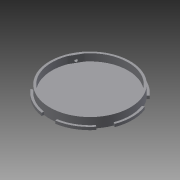
# Autodesk Inventor part: base
Saved by Autodesk Inventor 2015 (Build 190159000, 159)
## iProperties
Created: 2019-10-01
Part Number: base
Material: Generic
Document SubType Name: Modeling
Designer: gabri
Density: 1 g/cm^3
Appearance: Default
Author: gabri
Autodesk Inventor part; units mm, degrees
ref_plane "YZ Plane" through (0, 0, 0) normal (1, 0, 0) x (0, 1, 0)
sketch "Sketch1" plane through (0, 0, 0) normal (0, 0, 1) x (1, 0, 0)
  line L0 (-49.0069, -18.1093) -> (-50.1652, -19.0624) projected
  arc A0 (-50.1652, -19.0624) -> (-31.7077, -29.6283) centre (-27, 0) ccw projected
  line L1 (-31.7077, -29.6283) -> (-31.4723, -28.1469) projected
  arc A1 (-31.4723, -28.1469) -> (-22.3204, -28.1132) centre (-27, 0) ccw projected
  line L2 (-22.3204, -28.1132) -> (-22.0741, -29.5928) projected
  arc A2 (-22.0741, -29.5928) -> (-3.6949, -18.8911) centre (-27, 0) ccw projected
  line L3 (-3.6949, -18.8911) -> (-4.8602, -17.9466) projected
  arc A3 (-4.8602, -17.9466) -> (-0.3135, -10.0039) centre (-27, 0) ccw projected
  line L4 (-0.3135, -10.0039) -> (1.0911, -10.5304) projected
  arc A4 (1.0911, -10.5304) -> (1.0127, 10.7372) centre (-27, 0) ccw projected
  line L5 (1.0127, 10.7372) -> (-0.3879, 10.2004) projected
  arc A5 (-0.3879, 10.2004) -> (-4.9931, 18.1093) centre (-27, 0) ccw projected
  line L6 (-4.9931, 18.1093) -> (-3.8348, 19.0624) projected
  arc A6 (-3.8348, 19.0624) -> (-22.2923, 29.6283) centre (-27, 0) ccw projected
  line L7 (-22.2923, 29.6283) -> (-22.5277, 28.1469) projected
  arc A7 (-22.5277, 28.1469) -> (-31.6796, 28.1132) centre (-27, 0) ccw projected
  line L8 (-31.6796, 28.1132) -> (-31.9259, 29.5928) projected
  arc A8 (-31.9259, 29.5928) -> (-50.3051, 18.8911) centre (-27, 0) ccw projected
  line L9 (-50.3051, 18.8911) -> (-49.1398, 17.9466) projected
  arc A9 (-49.1398, 17.9466) -> (-53.6865, 10.0039) centre (-27, 0) ccw projected
  line L10 (-53.6865, 10.0039) -> (-55.0911, 10.5304) projected
  arc A10 (-55.0911, 10.5304) -> (-55.0127, -10.7372) centre (-27, 0) ccw projected
  line L11 (-55.0127, -10.7372) -> (-53.6121, -10.2004) projected
  arc A11 (-53.6121, -10.2004) -> (-49.0069, -18.1093) centre (-27, 0) ccw projected
  line L12 (-0.0417, 1.5) -> (1, 1.5) projected
  line L13 (1, 1.5) -> (1, -1.5) projected
  line L14 (1, -1.5) -> (-0.0417, -1.5) projected
  arc A12 (-53.9583, -1.5) -> (-0.0417, -1.5) centre (-27, 0) ccw projected
  line L15 (-53.9583, -1.5) -> (-55, -1.5) projected
  line L16 (-55, -1.5) -> (-55, 1.5) projected
  line L17 (-55, 1.5) -> (-53.9583, 1.5) projected
  arc A13 (-0.0417, 1.5) -> (-53.9583, 1.5) centre (-27, 0) ccw projected
  circle A14 centre (-27, 0) radius 30
  point P0 (0, 0)
  constraints: 1 centre point, 1 coincident, 1 concentric
extrude "Extrusion1" add sketch "Sketch1" along normal blind 2 contours A11 L11 A10 L10 A9 L9 A8 L8 A7 L7 A6 L6 A5 L5 A4 L4 A3 L3 A2 L2 A1 L1 A0 L0 | L12 L13 L14 A12 L15 L16 L17 A13
sketch "Sketch2" plane through (0, 0, 2) normal (0, 0, 1) x (1, 0, 0)
  arc A0 (-53.9583, -1.5) -> (-0.0417, -1.5) centre (-27, 0) ccw projected
  arc A1 (-0.0417, 1.5) -> (-53.9583, 1.5) centre (-27, 0) ccw projected
  circle A2 centre (-27, 0) radius 28.5 projected
  circle A3 centre (-27, 0) radius 27
  circle A4 centre (-27, 0) radius 28.5
  point P0 (0, 0)
  constraints: 2 centre point, 2 coincident, 2 concentric
ref_plane "Work Plane1" through (-31.9259, 28.1132, 7) normal (0, 0, 1) x (1, 0, 0)
extrude "Extrusion2" add sketch "Sketch2" along normal up to surface (5 mm away)
sketch "Sketch3" plane through (-27, 0, 2) normal (0, 0, 1) x (1, 0, 0)
  circle A0 centre (0, 0) radius 27 projected
  circle A1 centre (0, 0) radius 28.5 projected
  line L0 (-23.3051, 18.8911) -> (-28.0911, 10.5304) projected
  line L1 (-28.0911, 10.5304) -> (-26.6865, 10.0039) projected
  arc A2 (-22.1398, 17.9466) -> (-26.6865, 10.0039) centre (0, 0) ccw projected
  line L2 (-22.1398, 17.9466) -> (-23.3051, 18.8911) projected
  line L3 (-22.1398, 17.9466) -> (-20.9746, 17.002)
  line L4 (-26.6865, 10.0039) -> (-25.282, 9.4774)
  line L5 (-20.9746, 17.002) -> (-25.282, 9.4774)
  point P0 (27, 0)
  constraints: 6 end point, 2 collinear, 2 point on circle
ref_plane "Work Plane2" through (-55.0911, 10.0039, 7) normal (0, 0, 1) x (1, 0, 0)
extrude "Extrusion3" add sketch "Sketch3" along normal up to surface (5 mm away) contours L5 A0 picked at (-22.9781, 13.7109)
sketch "Sketch4" plane through (-52.282, 9.4774, 7) normal (0.8678623, -0.4968048, 0) x (0, 0, -1)
  circle A0 centre (2.5, 4.3351) radius 1 projected
  point P0 (7, 17.7489)
  constraints: 1 coincident
hole "Hole1" at (-50.1283, 13.2397, 4.5) direction (-0.8678623, 0.4968048, 0) diameter 2 depth 8 tip angle 118
pattern_circular "Circular Pattern1" count 6 over 360 about axis through (-27, 0, 2) along (0, 0, 1) of "Extrusion3", "Hole1"
sketch "Sketch5" plane through (0, 0, 2) normal (0, 0, 1) x (1, 0, 0)
  arc A0 (-52.282, 9.4774) -> (-52.2114, -9.6635) centre (-27, 0) ccw projected
  line L0 (-47.9746, 17.002) -> (-52.282, 9.4774) projected
  arc A1 (-31.4333, 26.6335) -> (-47.9746, 17.002) centre (-27, 0) ccw projected
  line L1 (-22.7631, 26.6655) -> (-31.4333, 26.6335) projected
  arc A2 (-6.1513, 17.1561) -> (-22.7631, 26.6655) centre (-27, 0) ccw projected
  line L2 (-1.7886, 9.6635) -> (-6.1513, 17.1561) projected
  arc A3 (-1.718, -9.4774) -> (-1.7886, 9.6635) centre (-27, 0) ccw projected
  line L3 (-6.0254, -17.002) -> (-1.718, -9.4774) projected
  arc A4 (-22.5667, -26.6335) -> (-6.0254, -17.002) centre (-27, 0) ccw projected
  line L4 (-31.2369, -26.6655) -> (-22.5667, -26.6335) projected
  arc A5 (-47.8487, -17.1561) -> (-31.2369, -26.6655) centre (-27, 0) ccw projected
  line L5 (-52.2114, -9.6635) -> (-47.8487, -17.1561) projected
  circle A6 centre (-27, 0) radius 28.5 projected
  line L6 (-53.6121, -10.2004) -> (-55.0127, -10.7372) projected
  line L7 (-55.0911, 10.5304) -> (-53.6865, 10.0039) projected
  line L8 (-53.6865, 10.0039) -> (-52.282, 9.4774)
  line L9 (-53.6121, -10.2004) -> (-52.2114, -9.6635)
  point P0 (0, 0)
  constraints: 4 end point, 2 collinear
extrude "Extrusion4" cut sketch "Sketch5" along normal up to surface (5 mm away) contours A0 L9 A6 L8
pattern_circular "Circular Pattern2" count 6 over 360 about axis through (-27, 0, 2) along (0, 0, 1) of "Extrusion4"
sketch "Sketch6" plane through (0, 0, 2) normal (0, 0, 1) x (1, 0, 0)
  line L0 (-53.6865, 10.0039) -> (-55.0911, 10.5304) projected
  arc A0 (-55.0911, 10.5304) -> (-55.0127, -10.7372) centre (-27, 0) ccw projected
  line L1 (-55.0127, -10.7372) -> (-53.6121, -10.2004) projected
  line L2 (-53.6121, -10.2004) -> (-52.2114, -9.6635) projected
  line L3 (-52.2114, -9.6635) -> (-47.8487, -17.1561) projected
  line L4 (-47.8487, -17.1561) -> (-49.0069, -18.1093) projected
  line L5 (-49.0069, -18.1093) -> (-50.1652, -19.0624) projected
  arc A1 (-50.1652, -19.0624) -> (-31.7077, -29.6283) centre (-27, 0) ccw projected
  line L6 (-31.7077, -29.6283) -> (-31.4723, -28.1469) projected
  line L7 (-31.4723, -28.1469) -> (-31.2369, -26.6655) projected
  line L8 (-31.2369, -26.6655) -> (-22.5667, -26.6335) projected
  line L9 (-22.5667, -26.6335) -> (-22.3204, -28.1132) projected
  line L10 (-22.3204, -28.1132) -> (-22.0741, -29.5928) projected
  arc A2 (-22.0741, -29.5928) -> (-3.6949, -18.8911) centre (-27, 0) ccw projected
  line L11 (-3.6949, -18.8911) -> (-4.8602, -17.9466) projected
  line L12 (-4.8602, -17.9466) -> (-6.0254, -17.002) projected
  line L13 (-6.0254, -17.002) -> (-1.718, -9.4774) projected
  line L14 (-1.718, -9.4774) -> (-0.3135, -10.0039) projected
  line L15 (-0.3135, -10.0039) -> (1.0911, -10.5304) projected
  arc A3 (1.0911, -10.5304) -> (1.0127, 10.7372) centre (-27, 0) ccw projected
  line L16 (1.0127, 10.7372) -> (-0.3879, 10.2004) projected
  line L17 (-0.3879, 10.2004) -> (-1.7886, 9.6635) projected
  line L18 (-1.7886, 9.6635) -> (-6.1513, 17.1561) projected
  line L19 (-6.1513, 17.1561) -> (-4.9931, 18.1093) projected
  line L20 (-4.9931, 18.1093) -> (-3.8348, 19.0624) projected
  arc A4 (-3.8348, 19.0624) -> (-22.2923, 29.6283) centre (-27, 0) ccw projected
  line L21 (-22.2923, 29.6283) -> (-22.5277, 28.1469) projected
  line L22 (-22.5277, 28.1469) -> (-22.7631, 26.6655) projected
  line L23 (-22.7631, 26.6655) -> (-31.4333, 26.6335) projected
  line L24 (-31.4333, 26.6335) -> (-31.6796, 28.1132) projected
  line L25 (-31.6796, 28.1132) -> (-31.9259, 29.5928) projected
  arc A5 (-31.9259, 29.5928) -> (-50.3051, 18.8911) centre (-27, 0) ccw projected
  line L26 (-50.3051, 18.8911) -> (-49.1398, 17.9466) projected
  line L27 (-49.1398, 17.9466) -> (-47.9746, 17.002) projected
  line L28 (-47.9746, 17.002) -> (-52.282, 9.4774) projected
  line L29 (-52.282, 9.4774) -> (-53.6865, 10.0039) projected
  arc A6 (-53.9583, -1.5) -> (-0.0417, -1.5) centre (-27, 0) ccw projected
  circle A7 centre (-27, 0) radius 27
  circle A8 centre (-27, 0) radius 30
  point P0 (0, 0)
  constraints: 2 centre point, 2 coincident, 2 concentric
extrude "Extrusion5" add sketch "Sketch6" along normal up to surface (5 mm away) contours L29 A7 A6 L2 L1 A0 L0 | L28 A7 L23 L18 A6 L13 L8 L3 | A5 L25 L24 A7 L27 L26 | L5 L4 A6 L7 L6 A1 | A4 L20 L19 A7 L22 L21 | L10 L9 A6 L12 L11 A2 | A3 L15 L14 A6 A7 L17 L16
sketch "Sketch7" plane through (-27, 0, 7) normal (0, 0, 1) x (0.8678623, -0.4968048, 0)
  arc A0 (22.6509, 14.6948) -> (-24.1413, -12.0912) centre (0, 0) ccw projected
  circle A1 centre (0, 0) radius 27
  point P0 (23.4323, 13.4137)
  constraints: 1 centre point, 1 coincident, 1 concentric
extrude "Extrusion6" cut sketch "Sketch7" against normal blind 5
sketch "Sketch8" plane through (-27, 0, 2) normal (0, 0, 1) x (1, 0, 0)
  line L0 (16, -16) -> (-16, -16)
  line L1 (-16, -16) -> (-16, 16)
  line L2 (-16, 16) -> (16, 16)
  line L3 (16, 16) -> (16, -16)
  line L4 (-17.5, -17.5) -> (17.5, -17.5)
  line L5 (17.5, -17.5) -> (17.5, 17.5)
  line L6 (17.5, 17.5) -> (-17.5, 17.5)
  line L7 (-17.5, 17.5) -> (-17.5, -17.5)
  line L8 (16, -16) -> (-16, 16)
  point P0 (27, 0)
  point P1 (0, 0)
  point P2 (0, 0)
  dimension "d25" = 32
  dimension "d26" = 32
  dimension "d27" = 1.5
  constraints: 18 end point, 4 parallel, 2 perpendicular, 1 horizontal, 1 midpoint, 3 other
  measures "d25" distance of L0.start L0.end
  measures "d26" distance of L0.end L1.end
  measures "d27" distance between parallel lines of L0 L4
extrude "Extrusion7" add sketch "Sketch8" along normal blind 6
sketch "Sketch9" plane through (-27, 0, 2) normal (0, 0, 1) x (1, 0, 0)
  circle A0 centre (0, 0) radius 27 projected
  circle A1 centre (0, -20) radius 1.85
  circle A2 centre (0, -20) radius 0.75
  line L0 (-17.5, -17.5) -> (17.5, -17.5) projected
  point P0 (27, 0)
  dimension "d31" = 3.7
  dimension "d32" = 1.5
  dimension "d33" = 2.5
  constraints: 2 centre point, 1 coincident, 1 horizontal alignment
  measures "d31" diameter of A1
  measures "d32" diameter of A2
  measures "d33" distance from line of L0 A1.centre
extrude "Extrusion8" add sketch "Sketch9" along normal blind 10 contours A1
pattern_circular "Circular Pattern3" count 4 over 360 about axis through (-27, 0, 7) along (0, 0, -1) of "Extrusion8"
sketch "Sketch10" plane through (-27, 0, 7) normal (0, 0, 1) x (0.8678623, -0.4968048, 0)
  circle A0 centre (0, 0) radius 27 projected
  arc A1 (-18.028, -22.0735) -> (-10.1022, -26.6495) centre (0, 0) ccw projected
  line L0 (-10.6339, -28.0521) -> (-10.1022, -26.6495) projected
  arc A2 (-10.6339, -28.0521) -> (10.6339, -28.0521) centre (0, 0) ccw projected
  line L1 (10.1022, -26.6495) -> (10.6339, -28.0521) projected
  arc A3 (10.1022, -26.6495) -> (18.028, -22.0735) centre (0, 0) ccw projected
  line L2 (18.9769, -23.2353) -> (18.028, -22.0735) projected
  arc A4 (18.9769, -23.2353) -> (29.6108, -4.8168) centre (0, 0) ccw projected
  line L3 (28.1302, -4.576) -> (29.6108, -4.8168) projected
  arc A5 (28.1302, -4.576) -> (28.1302, 4.576) centre (0, 0) ccw projected
  line L4 (29.6108, 4.8168) -> (28.1302, 4.576) projected
  arc A6 (29.6108, 4.8168) -> (18.9769, 23.2353) centre (0, 0) ccw projected
  line L5 (18.028, 22.0735) -> (18.9769, 23.2353) projected
  arc A7 (18.028, 22.0735) -> (10.1022, 26.6495) centre (0, 0) ccw projected
  line L6 (10.6339, 28.0521) -> (10.1022, 26.6495) projected
  arc A8 (10.6339, 28.0521) -> (-10.6339, 28.0521) centre (0, 0) ccw projected
  line L7 (-10.1022, 26.6495) -> (-10.6339, 28.0521) projected
  arc A9 (-10.1022, 26.6495) -> (-18.028, 22.0735) centre (0, 0) ccw projected
  line L8 (-18.9769, 23.2353) -> (-18.028, 22.0735) projected
  arc A10 (-18.9769, 23.2353) -> (-29.6108, 4.8168) centre (0, 0) ccw projected
  line L9 (-28.1302, 4.576) -> (-29.6108, 4.8168) projected
  arc A11 (-28.1302, 4.576) -> (-28.1302, -4.576) centre (0, 0) ccw projected
  line L10 (-29.6108, -4.8168) -> (-28.1302, -4.576) projected
  arc A12 (-29.6108, -4.8168) -> (-18.9769, -23.2353) centre (0, 0) ccw projected
  line L11 (-18.028, -22.0735) -> (-18.9769, -23.2353) projected
  line L12 (-5.2839, 30) -> (5.2839, 30)
  arc A13 (10.6339, 28.0521) -> (-10.6339, 28.0521) centre (0, 0) ccw projected
  line L13 (5.2097, 29.5442) -> (-5.2097, 29.5442)
  line L14 (-5.2839, 30) -> (-5.2036, 29.5442)
  line L15 (5.2036, 29.5442) -> (5.2839, 30)
  point P0 (23.4323, 13.4137)
  point P1 (0, 30)
  constraints: 8 end point, 3 point on circle, 2 point on line, 1 horizontal, 1 midpoint
extrude "Extrusion10" cut sketch "Sketch10" against normal blind 15 contours L14 L12 A8 | A8 L13 | L12 L15 A8
sketch "Sketch11" plane through (-27, 0, 7) normal (0, 0, 1) x (0.8641768, 0.5031884, 0)
  line L0 (28.1888, 10.266) -> (28.1878, 10.2656) projected
  line L1 (28.1878, 10.2656) -> (22.9842, 19.2785) projected
  line L2 (22.9842, 19.2785) -> (22.985, 19.2792) projected
  arc A0 (22.985, 19.2792) -> (18.9769, 23.2353) centre (0, 0) ccw projected
  line L3 (18.028, 22.0735) -> (18.9769, 23.2353) projected
  arc A1 (18.028, 22.0735) -> (10.1022, 26.6495) centre (0, 0) ccw projected
  line L4 (10.6339, 28.0521) -> (10.1022, 26.6495) projected
  arc A2 (10.6339, 28.0521) -> (-10.6339, 28.0521) centre (0, 0) ccw projected
  line L5 (-10.1022, 26.6495) -> (-10.6339, 28.0521) projected
  arc A3 (-10.1022, 26.6495) -> (-18.028, 22.0735) centre (0, 0) ccw projected
  line L6 (-18.9769, 23.2353) -> (-18.028, 22.0735) projected
  arc A4 (-18.9769, 23.2353) -> (-29.6108, 4.8168) centre (0, 0) ccw projected
  line L7 (-28.1302, 4.576) -> (-29.6108, 4.8168) projected
  arc A5 (-28.1302, 4.576) -> (-28.1302, -4.576) centre (0, 0) ccw projected
  line L8 (-29.6108, -4.8168) -> (-28.1302, -4.576) projected
  arc A6 (-29.6108, -4.8168) -> (-18.9769, -23.2353) centre (0, 0) ccw projected
  line L9 (-18.028, -22.0735) -> (-18.9769, -23.2353) projected
  arc A7 (-18.028, -22.0735) -> (-10.1022, -26.6495) centre (0, 0) ccw projected
  line L10 (-10.6339, -28.0521) -> (-10.1022, -26.6495) projected
  arc A8 (-10.6339, -28.0521) -> (10.6339, -28.0521) centre (0, 0) ccw projected
  line L11 (10.1022, -26.6495) -> (10.6339, -28.0521) projected
  arc A9 (10.1022, -26.6495) -> (18.028, -22.0735) centre (0, 0) ccw projected
  line L12 (18.9769, -23.2353) -> (18.028, -22.0735) projected
  arc A10 (18.9769, -23.2353) -> (29.6108, -4.8168) centre (0, 0) ccw projected
  line L13 (28.1302, -4.576) -> (29.6108, -4.8168) projected
  arc A11 (28.1302, -4.576) -> (28.1302, 4.576) centre (0, 0) ccw projected
  line L14 (29.6108, 4.8168) -> (28.1302, 4.576) projected
  arc A12 (29.6108, 4.8168) -> (28.1888, 10.266) centre (0, 0) ccw projected
  circle A13 centre (0, 0) radius 27 projected
  line L15 (28.1888, 10.266) -> (25.3699, 9.2394)
  line L16 (20.6865, 17.3513) -> (22.985, 19.2792)
  arc A14 (26.7794, 9.7527) -> (21.8358, 18.3153) centre (0, 0) ccw
  arc A15 (18.028, 22.0735) -> (28.1302, 4.576) centre (0, 0) ccw
  point P0 (23.3328, -13.5861)
  constraints: 6 end point, 6 point on circle, 2 centre point, 2 midpoint
extrude "Extrusion11" add sketch "Sketch11" along normal blind 7 contours L15 A14 L16 L1
sketch "Sketch12" plane through (-16.8383, 28.2255, 7) normal (0.4968048, 0.8678623, 0) x (0.8678623, -0.4968048, 0)
  line L0 (10.4072, -7) -> (0, -7) projected
  point P0 (28.6359, 7)
  point P1 (5.2036, -4)
  dimension "d49" = 3
  measures "d49" distance from line of L0 point (5.204, -4)
hole "Hole2" at (-12.3223, 25.6403, 11) direction (-0.4968048, -0.8678623, 0) diameter 2 depth 3 tip angle 118 countersink diameter 4 countersink angle 90
pattern_circular "Circular Pattern4" count 6 over 360 about axis through (-27, 0, 7) along (0, 0, -1) of "Hole2", "Extrusion11", "Extrusion10"
body "Solid1"
